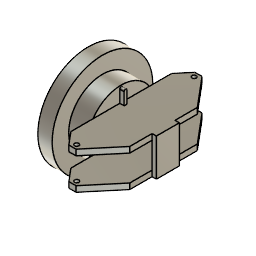
model (Autodesk Fusion 360 archive; units mm, degrees)
design "jaw 6"
part number: 2025-10-28-00-25-30-130
part number: 2025-10-28-00-26-21-145
Autodesk Fusion 360 part; units mm, degrees
sketch "Sketch1" plane through (0, 0, 0) normal (1, 0, 0) x (0, 1, 0)
  circle A0 centre (0, 0) radius 35
  dimension "d1" = 70
  constraint coincident A0.centre origin
  measures "d1" diameter of A0
extrude "Extrude1" add sketch "Sketch1" along normal blind 10 in component "Component"
sketch "Sketch2" plane through (10, 0, 0) normal (1, 0, 0) x (0, 1, 0)
  circle A0 centre (0, 0) radius 35
  circle A1 centre (0, 0) radius 23.5
  dimension "d4" = 47
  constraint concentric A0 A1
  measures "d4" diameter of A1
extrude "Extrude2" add sketch "Sketch2" along normal blind 13 contours A1 in component "Component"
ref_plane "WorkPlane1" through (0, 0, 13) normal (0, 0, 1) x (1, 0, 0)
sketch "Sketch3" plane through (0, 0, 13) normal (0, 0, 1) x (1, 0, 0)
  line L0 (23, 0) -> (23, -35)
  line L1 (23, -35) -> (23, -42)
  line L2 (23, -35) -> (30.3921, -43.8095)
  line L3 (30.3921, -43.8095) -> (35.3921, -43.8095)
  line L4 (23, 0) -> (63, 0)
  line L5 (23, -23.5) -> (65.3695, -23.5)
  line L6 (35.3921, -43.8095) -> (52.4338, -23.5)
  line L7 (35.3921, -43.8095) -> (49, -43.8095)
  line L8 (52.4338, -23.5) -> (52.4338, 0)
  line L9 (35.3921, 43.8095) -> (52.4338, 23.5)
  line L10 (30.3921, 43.8095) -> (35.3921, 43.8095)
  line L11 (23, 35) -> (30.3921, 43.8095)
  line L12 (23, 0) -> (23, 35)
  line L13 (23, 0) -> (63, 0)
  line L14 (52.4338, 23.5) -> (52.4338, 0)
  dimension "d8" = 35
  dimension "d9" = 11.5
  dimension "d10" = 40
  dimension "d11" = 5
  dimension "d12" = 50
  constraint vertical L0
  constraint parallel L0 L1
  constraint horizontal L3
  constraint perpendicular L0 L4
  constraint coincident L0 L5.start
  constraint perpendicular L0 L5
  constraint coincident L5 L6.end
  constraint parallel L3 L7
  constraint coincident L4 L8.end
  constraint perpendicular L4 L8
  constraint symmetric L0.start L4 L12.start
  constraint symmetric L0.end L4 L11.start
  constraint symmetric L2.end L4 L10.start
  constraint symmetric L3.end L4 L9.start
  constraint symmetric L13.end L4 L4.end
  constraint symmetric L4 L6.end L9.end
  constraint symmetric L4 L8.end L14.end
  measures "d8" distance of L0.start L0.end
  measures "d9" distance of L0.end L2.end
  measures "d10" angle of L1 L2
  measures "d11" distance of L2.end L3.end
  measures "d12" angle of L6 L7
extrude "Extrude3" add sketch "Sketch3" against normal blind 4 in component "Component"
sketch "Sketch4" plane through (0, 0, 13) normal (0, 0, 1) x (-1, 0, 0)
  line L0 (-23, -35) -> (-23, -19.5768)
  line L1 (-23, -19.5768) -> (-23, 19.5768)
  line L2 (-23, 19.5768) -> (-23, 35)
  line L3 (-23, 35) -> (-30.3921, 43.8095)
  line L4 (-30.3921, 43.8095) -> (-35.3921, 43.8095)
  line L5 (-35.3921, 43.8095) -> (-52.4338, 23.5)
  line L6 (-52.4338, 23.5) -> (-52.4338, -23.5)
  line L7 (-52.4338, -23.5) -> (-35.3921, -43.8095)
  line L8 (-35.3921, -43.8095) -> (-30.3921, -43.8095)
  line L9 (-30.3921, -43.8095) -> (-23, -35)
  line L10 (-32.8921, 43.8095) -> (-32.8921, 40.8095)
  circle A0 centre (-32.8921, 40.8095) radius 1.5
  dimension "d15" = 3
  dimension "d16" = 3
  constraint midpoint L4 L10.start
  constraint perpendicular L4 L10
  constraint coincident L10.end A0.centre
  measures "d15" distance of L10.start L10.end
  measures "d16" diameter of A0
extrude "Extrude4" cut sketch "Sketch4" against normal blind 11.5 contours A0 in component "Component"
mirror "Mirror1" about plane through (0, 0, 0) normal (0, 1, 0) of "Extrude4" in component "Component"
mirror "Mirror2" about plane through (0, 0, 0) normal (0, 0, 1) of "Extrude3", "Extrude4", "Mirror1" in component "Component"
sketch "Sketch5" plane through (23, 0, 0) normal (1, 0, 0) x (0, 1, 0)
  line L0 (-19.5768, 13) -> (19.5768, 13)
  arc A0 (19.5768, 13) -> (-19.5768, 13) centre (0, 0) ccw
  line L1 (0, 13) -> (0, 23.5)
  line L2 (0, 13) -> (-1, 13)
  line L3 (-1, 13) -> (-1, 13.5345)
  line L4 (-1, 13.5345) -> (-1, 22.5345)
  line L5 (-1, 22.5345) -> (1, 22.5345)
  line L6 (1, 22.5345) -> (1, 13)
  dimension "d23" = 1
  dimension "d24" = 9
  dimension "d25" = 2
  constraint midpoint L0 L1.start
  constraint midpoint A0 L1.end
  constraint perpendicular L1 L2
  constraint perpendicular L2 L3
  constraint perpendicular L2 L4
  constraint perpendicular L1 L5
  constraint coincident L0 L6.end
  constraint perpendicular L0 L6
  measures "d23" distance of L1.start L2.end
  measures "d24" distance of L3.end L4.end
  measures "d25" distance of L4.end L5.end
extrude "Extrude5" add sketch "Sketch5" along normal blind 3 contours L0 L1 L2 L3 L4 L5 | L0 L1 L5 L6 in component "Component"
fillet "Fillet1" radius 1 2 edges at (24.5, 1, 22.5345) (24.5, -1, 22.5345) in component "Component"
mirror "Mirror3" about plane through (0, 0, 0) normal (0, 0, 1) of "Extrude5", "Fillet1" in component "Component"
sketch "Sketch6" plane through (52.4338, 0, 0) normal (1, 0, 0) x (0, 1, 0)
  line L0 (23.5, 13) -> (-23.5, 13)
  line L1 (-23.5, 13) -> (-23.5, 9)
  line L2 (-23.5, 9) -> (23.5, 9)
  line L3 (23.5, 9) -> (23.5, 13)
  line L4 (8, -13) -> (-8, -13)
  line L5 (-8, -13) -> (-8, 13)
  line L6 (-8, 13) -> (8, 13)
  line L7 (8, 13) -> (8, -13)
  line L8 (8, -13) -> (-8, 13) construction
  line L9 (-8, -13) -> (8, 13) construction
  dimension "d32" = 16
  dimension "d33" = 26
  constraint horizontal L4
  constraint perpendicular L4 L5
  constraint parallel L4 L6
  constraint parallel L5 L7
  constraint coincident L8 origin
  constraint coincident L9 origin
  measures "d32" distance of L5.end L6.end
  measures "d33" distance of L4.end L5.end
extrude "Extrude6" add sketch "Sketch6" along normal blind 3 contours L0 L2 L5 L6 L7 | L2 L4 L5 L7 in component "Component"
sketch "Sketch7" plane through (0, 0, 0) normal (-1, 0, 0) x (0, -1, 0)
  circle A0 centre (0, 0) radius 35
  circle A1 centre (0, 0) radius 10
  dimension "d36" = 20
  constraint coincident A0.centre A1.centre
  measures "d36" diameter of A1
extrude "Extrude7" cut sketch "Sketch7" against normal blind 10 contours A1 in component "Component"
component "Component" placed x (1, 0, 0) y (0, 1, 0) z (0, 0, 1) at (0, 0, 0)
equation "d4 = 23.5 * 2 mm"

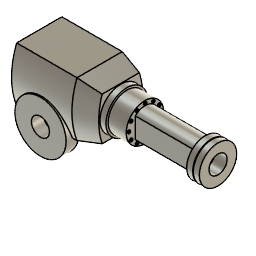
design "part 3"
part number: 2025-10-27-21-08-31-272
part number: 2025-10-27-21-14-58-809
Autodesk Fusion 360 part; units mm, degrees
sketch "Sketch1" plane through (0, 0, 0) normal (1, 0, 0) x (0, 1, 0)
  line L0 (0, 0) -> (0, 45)
  line L1 (0, 0) -> (0, -45)
  line L2 (0, 45) -> (37.5, 45)
  line L3 (0, 45) -> (-37.5, 45)
  line L4 (0, -45) -> (-37.5, -45)
  arc A0 (-37.5, 45) -> (-37.5, -45) centre (79.119, 0) ccw
  line L5 (0, -45) -> (37.5, -45)
  arc A1 (37.5, -45) -> (37.5, 45) centre (-79.119, 0) ccw
  dimension "d2" = 45
  dimension "d3" = 37.5
  dimension "d4" = 37.5
  dimension "d5" = 37.5
  dimension "d6" = 37.5
  dimension "d7" = 125
  dimension "d8" = 125
  constraint coincident L0.start L1.start
  constraint vertical L0
  constraint parallel L0 L1
  constraint perpendicular L0 L2
  constraint perpendicular L0 L3
  constraint perpendicular L1 L4
  constraint perpendicular L1 L5
  measures "d2" distance of L0.start L1.end
  measures "d3" distance of L0.end L2.end
  measures "d4" distance of L0.end L3.end
  measures "d5" distance of L1.end L4.end
  measures "d6" distance of L1.end L5.end
  measures "d7" radius of A1
  measures "d8" radius of A0
extrude "Extrude1" add sketch "Sketch1" along normal blind 100 in component "jaw 3"
extrude "Extrude2" add 1 faces at (100, -15.1807, 3.0661) along direction (1, 0, 0) blind 35 draft -15 in component "jaw 3"
sketch "Sketch2" plane through (135, 0, 0) normal (1, 0, 0) x (0, 1, 0)
  line L0 (-30.8786, -35.6218) -> (30.8786, -35.6218)
  arc A0 (30.8786, -35.6218) -> (30.8786, 35.6218) centre (-79.119, 0) ccw
  line L1 (30.8786, 35.6218) -> (-30.8786, 35.6218)
  arc A1 (-30.8786, 35.6218) -> (-30.8786, -35.6218) centre (79.119, 0) ccw
  circle A2 centre (0, 0) radius 34.5
  dimension "d13" = 69
  constraint coincident A2.centre origin
  measures "d13" diameter of A2
extrude "Extrude3" add sketch "Sketch2" along normal blind 10 contours A2 in component "jaw 3"
sketch "Sketch3" plane through (145, 0, 0) normal (1, 0, 0) x (0, 1, 0)
  circle A0 centre (0, 0) radius 34.5
  circle A1 centre (0, 0) radius 31
  dimension "d16" = 62
  constraint coincident A0.centre A1.centre
  measures "d16" diameter of A1
extrude "Extrude4" add sketch "Sketch3" along normal blind 30 contours A1 in component "jaw 3"
sketch "Sketch4" plane through (175, 0, 0) normal (1, 0, 0) x (0, 1, 0)
  circle A0 centre (0, 0) radius 31
  line L0 (0, 0) -> (27, 0)
  circle A1 centre (27, 0) radius 2.5
  circle A2 centre (27, 0) radius 1.5
  dimension "d19" = 27
  dimension "d20" = 5
  dimension "d21" = -1
  constraint coincident A0.centre L0.start
  constraint horizontal L0
  constraint coincident L0.end A1.centre
  measures "d19" distance of A0.centre L0.end
  measures "d20" diameter of A1
extrude "Extrude5" add sketch "Sketch4" along normal blind 1 contours A1 in component "jaw 3"
pattern_circular "C-Pattern1" count 12 over 360 about axis through (175, 0, 0) along (1, 0, 0) of "Extrude5" in component "jaw 3"
sketch "Sketch5" plane through (175, 0, 0) normal (1, 0, 0) x (0, 1, 0)
  circle A0 centre (13.5, -23.3827) radius 2.5
  circle A1 centre (-13.5, -23.3827) radius 2.5
  circle A2 centre (-27, 0) radius 2.5
  circle A3 centre (-13.5, 23.3827) radius 2.5
  circle A4 centre (13.5, 23.3827) radius 2.5
  circle A5 centre (27, 0) radius 2.5
  circle A6 centre (0, 0) radius 31
  circle A7 centre (23.3827, 13.5) radius 2.5
  circle A8 centre (0, 27) radius 2.5
  circle A9 centre (-23.3827, 13.5) radius 2.5
  circle A10 centre (-23.3827, -13.5) radius 2.5
  circle A11 centre (0, -27) radius 2.5
  circle A12 centre (23.3827, -13.5) radius 2.5
  line L0 (0, 0) -> (16, 0)
  line L1 (0, 0) -> (0, -6)
  line L2 (16, 0) -> (16, -17)
  line L3 (16, 0) -> (16, 17)
  line L4 (0, 0) -> (-16, 0)
  line L5 (-16, 0) -> (-16, -17)
  line L6 (-16, 0) -> (-16, 17)
  arc A13 (16, 17) -> (-16, 17) centre (0, 1.9003) ccw
  arc A14 (-16, -17) -> (16, -17) centre (0, -1.9003) ccw
  dimension "d26" = 16
  dimension "d27" = 17
  dimension "d28" = 17
  dimension "d29" = 16
  dimension "d30" = 17
  dimension "d31" = 17
  dimension "d32" = 22
  dimension "d33" = 22
  constraint coincident A6.centre L0.start
  constraint horizontal L0
  constraint perpendicular L0 L1
  constraint perpendicular L0 L2
  constraint perpendicular L0 L3
  constraint perpendicular L1 L4
  constraint perpendicular L4 L5
  constraint perpendicular L4 L6
  measures "d26" distance of A6.centre L0.end
  measures "d27" distance of L0.end L2.end
  measures "d28" distance of L0.end L3.end
  measures "d29" distance of A6.centre L4.end
  measures "d30" distance of L4.end L5.end
  measures "d31" distance of L4.end L6.end
  measures "d32" radius of A13
  measures "d33" radius of A14
extrude "Extrude6" add sketch "Sketch5" along normal blind 100 contours L0 L3 L4 L6 A13 | L0 L2 L4 L5 A14 in component "jaw 3"
sketch "Sketch6" plane through (275, 0, 0) normal (1, 0, 0) x (0, 1, 0)
  line L0 (-16, 17) -> (-16, -17)
  arc A0 (-16, -17) -> (16, -17) centre (0, -1.9003) ccw
  line L1 (16, -17) -> (16, 17)
  arc A1 (16, 17) -> (-16, 17) centre (0, 1.9003) ccw
  circle A2 centre (0, 0) radius 30.9959
  constraint coincident A2.centre origin
extrude "Extrude7" add sketch "Sketch6" along normal blind 10 contours L0 A0 L1 A1 | A2 in component "jaw 3"
sketch "Sketch7" plane through (285, 0, 0) normal (1, 0, 0) x (0, 1, 0)
  circle A0 centre (0, 0) radius 30.9959
  circle A1 centre (0, 0) radius 29.9959
  dimension "d38" = -1
extrude "Extrude8" add sketch "Sketch7" along normal blind 1 contours A1 in component "jaw 3"
sketch "Sketch8" plane through (286, 0, 0) normal (1, 0, 0) x (0, 1, 0)
  circle A0 centre (0, 0) radius 29.9959
  circle A1 centre (0, 0) radius 31.0015
  constraint coincident A0.centre A1.centre
extrude "Extrude9" add sketch "Sketch8" along normal blind 10 contours A0 | A1 in component "jaw 3"
ref_plane "WorkPlane1" through (0, -37.5, 45) normal (0, -1, 0) x (1, 0, 0)
sketch "Sketch9" plane through (0, -37.5, 0) normal (0, -1, 0) x (-1, 0, 0)
  circle A0 centre (-50, 45) radius 42.5
  dimension "d43" = 85
  measures "d43" diameter of A0
extrude "Extrude10" add sketch "Sketch9" along normal mid plane 21 in component "jaw 3"
sketch "Sketch10" plane through (0, -27, 0) normal (0, 1, 0) x (-1, 0, 0)
  line L0 (-7.5, -45) -> (-92.5, -45)
  arc A0 (-92.5, -45) -> (-7.5, -45) centre (-50, -45) ccw
  line L1 (-50, -45) -> (-50, -75)
  line L2 (-70, -45) -> (-70, -75.0144)
  line L3 (-30, -45) -> (-30, -75.0144)
  arc A1 (-70, -75.0144) -> (-30, -75.0144) centre (-50, -52.6537) ccw
  dimension "d46" = 30
  dimension "d47" = 20
  dimension "d48" = -20
  dimension "d49" = 30
  constraint coincident A0.centre L1.start
  constraint perpendicular L0 L1
  measures "d46" distance of A0.centre L1.end
  measures "d49" radius of A1
extrude "Extrude11" add sketch "Sketch10" along normal blind 35 contours L0 L2 L3 A1 in component "jaw 3"
sketch "Sketch11" plane through (70, 0, 0) normal (1, 0, 0) x (0, 1, 0)
  line L0 (-27, -45) -> (-27, -75.0144)
  line L1 (-27, -75.0144) -> (8, -75.0144)
  line L2 (8, -75.0144) -> (8, -45)
  line L3 (8, -45) -> (-27, -45)
  line L4 (8, -45) -> (33, -45)
  line L5 (8, -45) -> (8, -87)
  arc A0 (8, -87) -> (33, -45) centre (-21.8393, -40.7981) ccw
  dimension "d52" = 25
  dimension "d53" = 42
  dimension "d54" = 55
  constraint coincident L2.end L3.start
  constraint perpendicular L2 L4
  constraint perpendicular L1 L5
  measures "d52" distance of L2.end L4.end
  measures "d53" distance of L2.end L5.end
  measures "d54" radius of A0
extrude "Extrude12" add sketch "Sketch11" against normal blind 40 contours L2 L4 L5 A0 in component "jaw 3"
extrude "Extrude13" cut 1 faces at (50, 8, -85.5512) along direction (0, 1, 0) blind 90 in component "jaw 3"
sketch "Sketch12" plane through (296, 0, 0) normal (1, 0, 0) x (0, 1, 0)
  circle A0 centre (0, 0) radius 31.0015
  circle A1 centre (0, 0) radius 15
  dimension "d59" = 30
  constraint coincident A0.centre A1.centre
  measures "d59" diameter of A1
extrude "Extrude14" cut sketch "Sketch12" against normal blind 20 contours A1 in component "jaw 3"
sketch "Sketch13" plane through (0, -48, 0) normal (0, -1, 0) x (1, 0, 0)
  circle A0 centre (50, -45) radius 42.5
  circle A1 centre (50, -45) radius 15
  dimension "d62" = 30
  constraint concentric A0 A1
  measures "d62" diameter of A1
extrude "Extrude15" cut sketch "Sketch13" against normal blind 20 contours A1 in component "jaw 3"
component "jaw 3" placed x (1, 0, 0) y (0, 1, 0) z (0, 0, 1) at (0, 0, 0)
equation "d44 = ( 21 / 2 ) * 1 mm"

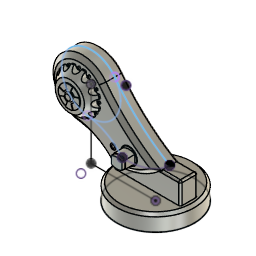
design "Jaw"
part number: 2025-10-27-12-31-22-567
part number: 2025-10-27-12-32-54-316
Autodesk Fusion 360 part; units mm, degrees
sketch "Sketch1" plane through (0, 0, 0) normal (0, 0, 1) x (1, 0, 0)
  circle A0 centre (0, 0) radius 90
  dimension "d1" = 180
  constraint coincident A0.centre origin
  measures "d1" diameter of A0
extrude "Extrude1" add sketch "Sketch1" along normal blind 37 in component "Component"
chamfer "Chamfer1" distance 6 angle 45 1 edges at (-83.9095, -32.5454, 37) in component "Component"
sketch "Sketch2" plane through (0, 0, 37) normal (0, 0, 1) x (-1, 0, 0)
  circle A0 centre (0, 0) radius 84
  line L0 (-77.5, 20) -> (77.5, 20)
  line L1 (77.5, 20) -> (77.5, -20)
  line L2 (77.5, -20) -> (-77.5, -20)
  line L3 (-77.5, -20) -> (-77.5, 20)
  line L4 (-77.5, 20) -> (77.5, -20) construction
  line L5 (77.5, 20) -> (-77.5, -20) construction
  dimension "d5" = 155
  dimension "d6" = 40
  constraint horizontal L0
  constraint perpendicular L0 L1
  constraint parallel L0 L2
  constraint parallel L1 L3
  constraint coincident L4 A0.centre
  constraint coincident L5 A0.centre
  constraint coincident A0.centre origin
  measures "d5" distance of L1.end L2.end
  measures "d6" distance of L0.end L1.end
  measures "d9" distance of L2.end
  measures "d10" distance of L2.end
extrude "Extrude2" add sketch "Sketch2" along normal blind 50 contours L0 L1 L2 L3 in component "Component"
sketch "Sketch3" plane through (0, -20, 0) normal (0, -1, 0) x (1, 0, 0)
  line L0 (-77.5, 37) -> (77.5, 37)
  line L1 (77.5, 37) -> (77.5, 87)
  line L2 (77.5, 87) -> (-77.5, 87)
  line L3 (-77.5, 87) -> (-77.5, 37)
  line L4 (-77.5, 87) -> (32.5, 87)
  line L5 (-77.5, 87) -> (-77.5, 48)
  arc A0 (-77.5, 48) -> (32.5, 87) centre (-68.6761, 197.7402) ccw
  dimension "d9" = 110
  dimension "d10" = 39
  dimension "d11" = 150
  constraint coincident L2.end L3.start
  constraint coincident L2 L4.end
  constraint coincident L3 L5.end
  measures "d9" distance of L2.end L4.end
  measures "d10" distance of L2.end L5.end
  measures "d11" radius of A0
extrude "Extrude3" cut sketch "Sketch3" against normal blind 230 contours L2 L3 L4 L5 A0 in component "Component"
sketch "Sketch4" plane through (0, 0, 0) normal (0, 1, 0) x (1, 0, 0)
  line L0 (0, 0) -> (-150, 0)
  circle A0 centre (-150, -160) radius 68.5
  arc A1 (32.5, -87) -> (-95.2795, -201.2057) centre (256.2101, -465.8849) ccw
  arc A2 (-158.3154, -92.0066) -> (-77.5, -48) centre (-173.4894, 32.069) ccw
  arc A3 (32.5, -87) -> (-77.5, -48) centre (-68.6761, -197.7402) ccw
  point P0 (-77.5, -48)
  point P1 (32.5, -87)
  dimension "d14" = 150
  dimension "d15" = 160
  dimension "d16" = 137
  dimension "d17" = 440
  dimension "d18" = 125
  dimension "d19" = 150
  constraint coincident L0.start origin
  constraint horizontal L0
  constraint tangent A0 A1
  constraint tangent A0 A2
  constraint coincident P0 A2.end
  constraint coincident P1 A1.start
  constraint coincident A0 A1.end
  constraint coincident A0 A2.start
  measures "d14" distance of L0.start L0.end
  measures "d15" distance of L0.end A0.centre
  measures "d16" diameter of A0
  measures "d17" radius of A1
  measures "d18" radius of A2
  measures "d19" radius of A3
extrude "Extrude4" add sketch "Sketch4" along normal mid plane 40 in component "Component"
sketch "Sketch5" plane through (0, 0, 0) normal (0, 1, 0) x (1, 0, 0)
  circle A0 centre (-150, -160) radius 68.5
  arc A1 (32.5, -87) -> (-95.2795, -201.2057) centre (256.2101, -465.8849) ccw
  arc A2 (-158.3154, -92.0066) -> (-77.5, -48) centre (-173.4894, 32.069) ccw
  arc A3 (32.5, -87) -> (-77.5, -48) centre (-68.6761, -197.7402) ccw
  line L0 (-150, -160) -> (-150, 0)
  constraint coincident A0.centre L0.start
  constraint vertical L0
sketch "Sketch6" plane through (0, -20, 0) normal (0, -1, 0) x (1, 0, 0)
  line L0 (-77.5, 48) -> (-77.5, 37)
  line L1 (-77.5, 37) -> (77.5, 37)
  line L2 (77.5, 37) -> (77.5, 87)
  line L3 (77.5, 87) -> (32.5, 87)
  arc A0 (-95.2795, 201.2057) -> (32.5, 87) centre (256.2101, 465.8849) ccw
  arc A1 (-95.2795, 201.2057) -> (-158.3154, 92.0066) centre (-150, 160) ccw
  arc A2 (-77.5, 48) -> (-158.3154, 92.0066) centre (-173.4894, -32.069) ccw
  arc A3 (-95.2795, 201.2057) -> (32.5, 87) centre (256.2101, 465.8849) ccw
  arc A4 (-77.5, 48) -> (-158.3154, 92.0066) centre (-173.4894, -32.069) ccw
  circle A5 centre (-150, 160) radius 68.5
  arc A6 (-77.5, 48) -> (32.5, 87) centre (-68.6761, 197.7402) ccw
extrude "Extrude5" add sketch "Sketch6" along normal blind 7.5 draft -55 contours A0 A2 A3 A4 A5 A6 | A1 A5 in component "Component"
sketch "Sketch7" plane through (0, -27.5, 0) normal (0, -1, 0) x (1, 0, 0)
  arc A0 (-103.8359, 194.7625) -> (-157.0151, 102.6385) centre (-150, 160) ccw
  arc A1 (-72.4228, 58.5017) -> (-157.0151, 102.6385) centre (-173.4894, -32.069) ccw
  arc A2 (-72.4228, 58.5017) -> (14.1053, 85.7195) centre (-68.6761, 197.7402) ccw
  arc A3 (-103.8359, 194.7625) -> (14.1053, 85.7195) centre (256.2101, 465.8849) ccw
  circle A4 centre (-150, 160) radius 50
  dimension "d24" = 100
  constraint concentric A0 A4
  measures "d24" diameter of A4
extrude "Extrude6" add sketch "Sketch7" along normal blind 3 contours A4 in component "Component"
extrude "Extrude7" add 1 faces at (-167.3965, -30.5, 167.9656) along direction (0, -1, 0) blind 19 draft -40 in component "Component"
sketch "Sketch8" plane through (0, -49.5, 0) normal (0, -1, 0) x (1, 0, 0)
  circle A0 centre (-150, 160) radius 34.0571
  line L0 (-150, 160) -> (-150, 210)
  arc A1 (-158.9635, 209.19) -> (-150, 201) centre (-150, 210) ccw
  circle A2 centre (-150, 160) radius 50
  arc A3 (-150, 201) -> (-141.0365, 209.19) centre (-150, 210) ccw
  dimension "d29" = 9
  dimension "d30" = 9
  constraint coincident A0.centre L0.start
  constraint vertical L0
  constraint coincident L0 A1.end
  constraint coincident A1.start A2
  constraint symmetric L0 A1.end A3.start
  constraint symmetric L0 A1.start A3.end
  constraint symmetric L0 A1 A3
  measures "d29" distance of L0.end A1.end
  measures "d30" radius of A1
extrude "Extrude8" cut sketch "Sketch8" against normal up to surface (22 mm away) contours L0 A1 A2 | L0 A2 A3 in component "Component"
sketch "Sketch9" plane through (0, -27.5, 0) normal (0, -1, 0) x (1, 0, 0)
  arc A0 (-158.9635, 209.19) -> (-141.0365, 209.19) centre (-150, 160) ccw
  arc A1 (-158.9635, 209.19) -> (-141.0365, 209.19) centre (-150, 210) ccw
  arc A2 (-103.8359, 194.7625) -> (-157.0151, 102.6385) centre (-150, 160) ccw
  arc A3 (-72.4228, 58.5017) -> (-157.0151, 102.6385) centre (-173.4894, -32.069) ccw
  arc A4 (-72.4228, 58.5017) -> (14.1053, 85.7195) centre (-68.6761, 197.7402) ccw
  arc A5 (-103.8359, 194.7625) -> (14.1053, 85.7195) centre (256.2101, 465.8849) ccw
  line L0 (-150, 201) -> (-150, 217.7889)
  circle A6 centre (-150, 207) radius 3
  circle A7 centre (-150, 207) radius 1.6
  dimension "d33" = 6
  dimension "d34" = -1.4
  constraint midpoint A1 L0.start
  constraint coincident A2 L0.end
  constraint vertical L0
  constraint coincident L0 A6.centre
  measures "d33" diameter of A6
extrude "Extrude9" add sketch "Sketch9" along normal blind 3 contours L0 A6 A7 | L0 A6 A7 in component "Component"
pattern_circular "C-Pattern1" count 12 over 360 about axis through (-150, -49.5, 160) along (0, 1, 0) of "Extrude8", "Extrude9" in component "Component"
sketch "Sketch10" plane through (0, -49.5, 0) normal (0, -1, 0) x (1, 0, 0)
  circle A0 centre (-150, 160) radius 34.0571
  circle A1 centre (-150, 160) radius 13
  circle A2 centre (-150, 160) radius 25
  dimension "d39" = 26
  dimension "d40" = 50
  constraint concentric A0 A1
  constraint concentric A1 A2
  measures "d39" diameter of A1
  measures "d40" diameter of A2
extrude "Extrude10" add sketch "Sketch10" along normal blind 1 contours A1 | A2 in component "Component"
sketch "Sketch11" plane through (0, -50.5, 0) normal (0, -1, 0) x (1, 0, 0)
  circle A0 centre (-150, 160) radius 25
  circle A1 centre (-150, 160) radius 12.5
  line L0 (-154.799, 171.5421) -> (-159.0764, 183.2942)
  line L1 (-146.3157, 171.9447) -> (-141.6715, 183.5719)
  line L2 (-161.5421, 155.201) -> (-173.2942, 150.9236)
  line L3 (-161.9447, 163.6843) -> (-173.5719, 168.3285)
  line L4 (-145.201, 148.4579) -> (-140.9236, 136.7058)
  line L5 (-153.6843, 148.0553) -> (-158.3285, 136.4281)
  line L6 (-138.4579, 164.799) -> (-126.7058, 169.0764)
  line L7 (-138.0553, 156.3157) -> (-126.4281, 151.6715)
  dimension "d43" = 25
  dimension "d46" = 360
  constraint concentric A0 A1
  constraint coincident A1 L0.start
  constraint coincident A0 L0.end
  constraint coincident A0 L1.end
  constraint coincident A1 L1.start
  measures "d43" diameter of A1
extrude "Extrude11" add sketch "Sketch11" along normal blind 1 contours A0 A1 L6 L7 | A0 A1 L0 L1 | A1 | A0 A1 L4 L5 | A0 A1 L2 L3 in component "Component"
sketch "Sketch12" plane through (0, -51.5, 0) normal (0, -1, 0) x (1, 0, 0)
  arc A0 (-145.201, 148.4579) -> (-138.0553, 156.3157) centre (-150, 160) ccw
  line L0 (-138.0553, 156.3157) -> (-126.4281, 151.6715)
  arc A1 (-126.4281, 151.6715) -> (-126.7058, 169.0764) centre (-150, 160) ccw
  line L1 (-126.7058, 169.0764) -> (-138.4579, 164.799)
  arc A2 (-138.4579, 164.799) -> (-146.3157, 171.9447) centre (-150, 160) ccw
  line L2 (-146.3157, 171.9447) -> (-141.6715, 183.5719)
  arc A3 (-141.6715, 183.5719) -> (-159.0764, 183.2942) centre (-150, 160) ccw
  line L3 (-159.0764, 183.2942) -> (-154.799, 171.5421)
  arc A4 (-154.799, 171.5421) -> (-161.9447, 163.6843) centre (-150, 160) ccw
  line L4 (-161.9447, 163.6843) -> (-173.5719, 168.3285)
  arc A5 (-173.5719, 168.3285) -> (-173.2942, 150.9236) centre (-150, 160) ccw
  line L5 (-173.2942, 150.9236) -> (-161.5421, 155.201)
  arc A6 (-161.5421, 155.201) -> (-153.6843, 148.0553) centre (-150, 160) ccw
  line L6 (-153.6843, 148.0553) -> (-158.3285, 136.4281)
  arc A7 (-158.3285, 136.4281) -> (-140.9236, 136.7058) centre (-150, 160) ccw
  line L7 (-140.9236, 136.7058) -> (-145.201, 148.4579)
  circle A8 centre (-150, 160) radius 9.5
  dimension "d49" = 19
  constraint concentric A0 A8
  measures "d49" diameter of A8
extrude "Extrude12" add sketch "Sketch12" along normal blind 3 draft -45 contours A8 in component "Component"
sketch "Sketch13" plane through (0, -27.5, 0) normal (0, -1, 0) x (1, 0, 0)
  circle A0 centre (-190.7032, 183.5) radius 3
  circle A1 centre (-190.7032, 136.5) radius 3
  circle A2 centre (-150, 113) radius 3
  circle A3 centre (-109.2968, 136.5) radius 3
  circle A4 centre (-109.2968, 183.5) radius 3
  circle A5 centre (-150, 207) radius 3
  arc A6 (-133.1676, 207.0815) -> (-141.0365, 209.19) centre (-150, 160) ccw
  arc A7 (-133.1676, 207.0815) -> (-117.6424, 198.118) centre (-125, 203.3013) ccw
  arc A8 (-111.8819, 192.3576) -> (-117.6424, 198.1181) centre (-150, 160) ccw
  arc A9 (-111.8819, 192.3576) -> (-102.9185, 176.8324) centre (-106.6987, 185) ccw
  arc A10 (-100.81, 168.9635) -> (-102.9185, 176.8324) centre (-150, 160) ccw
  arc A11 (-100.81, 168.9635) -> (-100.81, 151.0365) centre (-100, 160) ccw
  arc A12 (-102.9185, 143.1676) -> (-100.81, 151.0365) centre (-150, 160) ccw
  arc A13 (-102.9185, 143.1676) -> (-111.882, 127.6424) centre (-106.6987, 135) ccw
  arc A14 (-117.6424, 121.8819) -> (-111.8819, 127.6424) centre (-150, 160) ccw
  arc A15 (-117.6424, 121.8819) -> (-133.1676, 112.9185) centre (-125, 116.6987) ccw
  arc A16 (-141.0365, 110.81) -> (-133.1676, 112.9185) centre (-150, 160) ccw
  arc A17 (-141.0365, 110.81) -> (-158.9635, 110.81) centre (-150, 110) ccw
  arc A18 (-166.8324, 112.9185) -> (-158.9635, 110.81) centre (-150, 160) ccw
  arc A19 (-166.8324, 112.9185) -> (-182.3576, 121.882) centre (-175, 116.6987) ccw
  arc A20 (-188.1181, 127.6424) -> (-182.3576, 121.8819) centre (-150, 160) ccw
  arc A21 (-188.1181, 127.6424) -> (-197.0815, 143.1676) centre (-193.3013, 135) ccw
  arc A22 (-199.19, 151.0365) -> (-197.0815, 143.1676) centre (-150, 160) ccw
  arc A23 (-199.19, 151.0365) -> (-199.19, 168.9635) centre (-200, 160) ccw
  arc A24 (-197.0815, 176.8324) -> (-199.19, 168.9635) centre (-150, 160) ccw
  arc A25 (-197.0815, 176.8324) -> (-188.118, 192.3576) centre (-193.3013, 185) ccw
  arc A26 (-182.3576, 198.1181) -> (-188.1181, 192.3576) centre (-150, 160) ccw
  arc A27 (-182.3576, 198.1181) -> (-166.8324, 207.0815) centre (-175, 203.3013) ccw
  arc A28 (-158.9635, 209.19) -> (-166.8324, 207.0815) centre (-150, 160) ccw
  arc A29 (-158.9635, 209.19) -> (-141.0365, 209.19) centre (-150, 210) ccw
  arc A30 (-103.8359, 194.7625) -> (-157.0151, 102.6385) centre (-150, 160) ccw
  arc A31 (-72.4228, 58.5017) -> (-157.0151, 102.6385) centre (-173.4894, -32.069) ccw
  arc A32 (-72.4228, 58.5017) -> (14.1053, 85.7195) centre (-68.6761, 197.7402) ccw
  arc A33 (-103.8359, 194.7625) -> (14.1053, 85.7195) centre (256.2101, 465.8849) ccw
  circle A34 centre (-126.5, 200.7032) radius 3
  circle A35 centre (-103, 160) radius 3
  circle A36 centre (-126.5, 119.2968) radius 3
  circle A37 centre (-173.5, 119.2968) radius 3
  circle A38 centre (-197, 160) radius 3
  circle A39 centre (-173.5, 200.7032) radius 3
  line L0 (-47.7688, 96.5857) -> (-20.7688, 96.5857)
  line L1 (-20.7688, 96.5857) -> (-20.7688, 77.5857)
  line L2 (-20.7688, 77.5857) -> (-47.7688, 77.5857)
  line L3 (-47.7688, 77.5857) -> (-47.7688, 96.5857)
  arc A40 (-20.7688, 96.5857) -> (-47.7688, 96.5857) centre (-34.2688, 73.203) ccw
  arc A41 (-47.7688, 77.5857) -> (-20.7688, 77.5857) centre (-34.2688, 100.9684) ccw
  dimension "d52" = 27
  dimension "d53" = 19
  dimension "d54" = 27
  dimension "d55" = 27
  constraint horizontal L0
  constraint vertical L1
  constraint horizontal L2
  constraint vertical L3
  measures "d52" distance of L0.start L0.end
  measures "d53" distance of L0.start L2.end
  measures "d54" radius of A40
  measures "d55" radius of A41
extrude "Extrude13" add sketch "Sketch13" along normal blind 22 contours L0 A40 | L0 L1 L2 L3 | L2 A41 in component "Component"
sketch "Sketch14" plane through (0, -49.5, 0) normal (0, -1, 0) x (1, 0, 0)
  arc A0 (-20.7688, 96.5857) -> (-47.7688, 96.5857) centre (-34.2688, 73.203) ccw
  line L0 (-47.7688, 96.5857) -> (-47.7688, 77.5857)
  arc A1 (-47.7688, 77.5857) -> (-20.7688, 77.5857) centre (-34.2688, 100.9684) ccw
  line L1 (-20.7688, 77.5857) -> (-20.7688, 96.5857)
  arc A2 (-46.6178, 78.26) -> (-21.9198, 78.26) centre (-34.2688, 100.9684) ccw
  line L2 (-21.9198, 78.26) -> (-21.9198, 95.9115)
  arc A3 (-21.9198, 95.9115) -> (-46.6178, 95.9115) centre (-34.2688, 73.203) ccw
  line L3 (-46.6178, 95.9115) -> (-46.6178, 78.26)
  dimension "d58" = -1.151
extrude "Extrude14" add sketch "Sketch14" along normal blind 7 contours A2 L2 A3 L3 in component "Component"
sketch "Sketch15" plane through (0, -56.5, 0) normal (0, -1, 0) x (1, 0, 0)
  line L0 (-46.6178, 95.9115) -> (-46.6178, 78.26)
  arc A0 (-46.6178, 78.26) -> (-21.9198, 78.26) centre (-34.2688, 100.9684) ccw
  line L1 (-21.9198, 78.26) -> (-21.9198, 95.9115)
  arc A1 (-21.9198, 95.9115) -> (-46.6178, 95.9115) centre (-34.2688, 73.203) ccw
sketch "Sketch16" plane through (0, -27.5, 0) normal (0, -1, 0) x (1, 0, 0)
  line L0 (-20.7688, 96.5857) -> (-20.7688, 77.5857)
  arc A0 (-47.7688, 77.5857) -> (-20.7688, 77.5857) centre (-34.2688, 100.9684) ccw
  line L1 (-47.7688, 77.5857) -> (-47.7688, 96.5857)
  arc A1 (-20.7688, 96.5857) -> (-47.7688, 96.5857) centre (-34.2688, 73.203) ccw
  circle A2 centre (-190.7032, 183.5) radius 3
  circle A3 centre (-190.7032, 136.5) radius 3
  circle A4 centre (-150, 113) radius 3
  circle A5 centre (-109.2968, 136.5) radius 3
  circle A6 centre (-109.2968, 183.5) radius 3
  circle A7 centre (-150, 207) radius 3
  arc A8 (-133.1676, 207.0815) -> (-141.0365, 209.19) centre (-150, 160) ccw
  arc A9 (-133.1676, 207.0815) -> (-117.6424, 198.118) centre (-125, 203.3013) ccw
  arc A10 (-111.8819, 192.3576) -> (-117.6424, 198.1181) centre (-150, 160) ccw
  arc A11 (-111.8819, 192.3576) -> (-102.9185, 176.8324) centre (-106.6987, 185) ccw
  arc A12 (-100.81, 168.9635) -> (-102.9185, 176.8324) centre (-150, 160) ccw
  arc A13 (-100.81, 168.9635) -> (-100.81, 151.0365) centre (-100, 160) ccw
  arc A14 (-102.9185, 143.1676) -> (-100.81, 151.0365) centre (-150, 160) ccw
  arc A15 (-102.9185, 143.1676) -> (-111.882, 127.6424) centre (-106.6987, 135) ccw
  arc A16 (-117.6424, 121.8819) -> (-111.8819, 127.6424) centre (-150, 160) ccw
  arc A17 (-117.6424, 121.8819) -> (-133.1676, 112.9185) centre (-125, 116.6987) ccw
  arc A18 (-141.0365, 110.81) -> (-133.1676, 112.9185) centre (-150, 160) ccw
  arc A19 (-141.0365, 110.81) -> (-158.9635, 110.81) centre (-150, 110) ccw
  arc A20 (-166.8324, 112.9185) -> (-158.9635, 110.81) centre (-150, 160) ccw
  arc A21 (-166.8324, 112.9185) -> (-182.3576, 121.882) centre (-175, 116.6987) ccw
  arc A22 (-188.1181, 127.6424) -> (-182.3576, 121.8819) centre (-150, 160) ccw
  arc A23 (-188.1181, 127.6424) -> (-197.0815, 143.1676) centre (-193.3013, 135) ccw
  arc A24 (-199.19, 151.0365) -> (-197.0815, 143.1676) centre (-150, 160) ccw
  arc A25 (-199.19, 151.0365) -> (-199.19, 168.9635) centre (-200, 160) ccw
  arc A26 (-197.0815, 176.8324) -> (-199.19, 168.9635) centre (-150, 160) ccw
  arc A27 (-197.0815, 176.8324) -> (-188.118, 192.3576) centre (-193.3013, 185) ccw
  arc A28 (-182.3576, 198.1181) -> (-188.1181, 192.3576) centre (-150, 160) ccw
  arc A29 (-182.3576, 198.1181) -> (-166.8324, 207.0815) centre (-175, 203.3013) ccw
  arc A30 (-158.9635, 209.19) -> (-166.8324, 207.0815) centre (-150, 160) ccw
  arc A31 (-158.9635, 209.19) -> (-141.0365, 209.19) centre (-150, 210) ccw
  arc A32 (-103.8359, 194.7625) -> (-157.0151, 102.6385) centre (-150, 160) ccw
  arc A33 (-72.4228, 58.5017) -> (-157.0151, 102.6385) centre (-173.4894, -32.069) ccw
  arc A34 (-72.4228, 58.5017) -> (14.1053, 85.7195) centre (-68.6761, 197.7402) ccw
  arc A35 (-103.8359, 194.7625) -> (14.1053, 85.7195) centre (256.2101, 465.8849) ccw
  circle A36 centre (-126.5, 200.7032) radius 3
  circle A37 centre (-103, 160) radius 3
  circle A38 centre (-126.5, 119.2968) radius 3
  circle A39 centre (-173.5, 119.2968) radius 3
  circle A40 centre (-197, 160) radius 3
  circle A41 centre (-173.5, 200.7032) radius 3
  line L2 (-47.7688, 77.5857) -> (-20.7688, 96.5857)
  circle A42 centre (-34.2688, 87.0857) radius 17.857
  circle A43 centre (-34.2688, 87.0857) radius 19.1735
  circle A44 centre (-71.2492, 87.0857) radius 6.5
  circle A45 centre (-71.2492, 87.0857) radius 3.5
  dimension "d61" = 35.714
  dimension "d62" = 38.347
  dimension "d63" = 13
  dimension "d64" = 7
  constraint coincident L0.start A1.start
  constraint coincident A0.start L1.start
  constraint midpoint L2 A42.centre
  constraint concentric A42 A43
  constraint concentric A44 A45
  measures "d61" diameter of A42
  measures "d62" diameter of A43
  measures "d63" diameter of A44
  measures "d64" diameter of A45
extrude "Extrude15" cut sketch "Sketch16" against normal blind 0.9 contours A43 | A44 in component "Component"
sketch "Sketch17" plane through (0, 0, 0) normal (0, 0, 1) x (1, 0, 0)
  circle A0 centre (0, 0) radius 15
  dimension "d67" = 30
  constraint coincident A0.centre origin
  measures "d67" diameter of A0
extrude "Extrude16" cut sketch "Sketch17" along normal blind 20 in component "Component"
fillet "Fillet1" radius 4 10 edges at (77.5, 20, 62) (55, 20, 87) (-113.7109, 20, 77.7105) (-209.3252, 20, 194.2458) (-37.0038, 20, 137.8215) (77.5, 0, 87) (77.5, -20, 62) (55, -20, 87) (-77.5, -20, 42.5) (-77.5, 20, 42.5) in component "Component"
sketch "Sketch18" plane through (0, 20, 0) normal (0, 1, 0) x (-1, 0, 0)
  line L0 (-73.5, 83) -> (-73.5, 37)
  line L1 (-73.5, 37) -> (73.5, 37)
  line L2 (73.5, 37) -> (73.5, 49.4364)
  arc A0 (157.8298, 95.977) -> (73.5, 49.4364) centre (173.4894, -32.069) ccw
  arc A1 (157.8298, 95.977) -> (98.4748, 198.7996) centre (150, 160) ccw
  arc A2 (-31.4099, 83) -> (98.4748, 198.7996) centre (-256.2101, 465.8849) ccw
  line L3 (-31.4099, 83) -> (-73.5, 83)
  circle A3 centre (150, 160) radius 15
  dimension "d72" = 30
  constraint concentric A1 A3
  measures "d72" diameter of A3
extrude "Extrude17" cut sketch "Sketch18" against normal blind 20 contours A3 in component "Component"
component "Component" placed x (1, 0, 0) y (0, 1, 0) z (0, 0, 1) at (0, 0, 0)

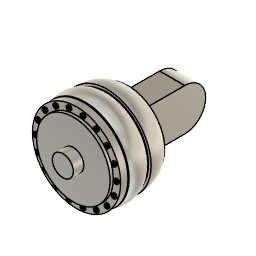
design "industrial bot"
part number: 2025-10-27-23-58-21-680
Autodesk Fusion 360 part; units mm, degrees
sketch "Sketch1" plane through (0, 0, 0) normal (0, 0, 1) x (1, 0, 0)
  line L0 (0, 0) -> (-35, 0)
  line L1 (0, 0) -> (0, -20)
  line L2 (0, -20) -> (-42, -20)
  arc A0 (-35, 0) -> (-42, -20) centre (-17.1273, -17.4804) ccw
  dimension "d1" = 35
  dimension "d2" = 20
  dimension "d3" = 42
  dimension "d4" = 25
  constraint coincident L0.start L1.start
  constraint horizontal L0
  constraint perpendicular L0 L1
  constraint perpendicular L1 L2
  measures "d1" distance of L0.start L0.end
  measures "d2" distance of L0.start L1.end
  measures "d3" distance of L1.end L2.end
  measures "d4" radius of A0
revolve "Revolve1" add sketch "Sketch1" angle 360 about axis through (0, 0, 0) along (0, -1, 0) makes body 1
sketch "Sketch2" plane through (0, -20, 0) normal (0, -1, 0) x (1, 0, 0)
  circle A0 centre (0, 0) radius 42
  circle A1 centre (0, 0) radius 39.5
  dimension "d6" = 79
  constraint coincident A0.centre A1.centre
  measures "d6" diameter of A1
extrude "Extrude1" add sketch "Sketch2" along normal blind 1 contours A1 bodies 1
sketch "Sketch3" plane through (0, 0, 0) normal (0, 0, 1) x (1, 0, 0)
  line L0 (0, -21) -> (0, -41)
  line L1 (0, -41) -> (-42, -41)
  line L2 (0, -21) -> (-40, -21)
  arc A0 (-40, -21) -> (-42, -41) centre (-23.7942, -32.7206) ccw
  dimension "d9" = 20
  dimension "d10" = 42
  dimension "d11" = 40
  dimension "d12" = 20
  constraint vertical L0
  constraint perpendicular L0 L1
  constraint perpendicular L0 L2
  measures "d9" distance of L0.start L0.end
  measures "d10" distance of L0.end L1.end
  measures "d11" distance of L0.start L2.end
  measures "d12" radius of A0
revolve "Revolve2" add sketch "Sketch3" angle 360 about axis through (0, -21, 0) along (0, -1, 0) bodies 1
sketch "Sketch4" plane through (0, -41, 0) normal (0, -1, 0) x (1, 0, 0)
  circle A0 centre (0, 0) radius 42
  circle A1 centre (0, 0) radius 41.25
  dimension "d14" = 82.5
  constraint coincident A0.centre A1.centre
  measures "d14" diameter of A1
extrude "Extrude2" add sketch "Sketch4" along normal blind 1 contours A1 bodies 1
sketch "Sketch5" plane through (0, -42, 0) normal (0, -1, 0) x (1, 0, 0)
  circle A0 centre (0, 0) radius 41.25
  circle A1 centre (0, 0) radius 42
  dimension "d17" = 84
  constraint coincident A0.centre A1.centre
  measures "d17" diameter of A1
extrude "Extrude3" add sketch "Sketch5" along normal blind 7 contours A0 | A1 bodies 1
sketch "Sketch6" plane through (0, -49, 0) normal (0, -1, 0) x (1, 0, 0)
  circle A0 centre (0, 0) radius 42
  circle A1 centre (0, 0) radius 35
  dimension "d20" = 70
  constraint coincident A0.centre A1.centre
  measures "d20" diameter of A1
extrude "Extrude4" add sketch "Sketch6" along normal blind 3 contours A1 bodies 1
sketch "Sketch7" plane through (0, -52, 0) normal (0, -1, 0) x (1, 0, 0)
  circle A0 centre (0, 0) radius 35
  line L0 (0, 0) -> (35, 0)
  line L1 (35, 0) -> (42, 0)
  circle A1 centre (38.5, 0) radius 2.25
  circle A2 centre (38.5, 0) radius 1.5
  dimension "d23" = 4.5
  dimension "d24" = 3
  constraint coincident A0.centre L0.start
  constraint coincident A0 L0.end
  constraint horizontal L0
  constraint parallel L0 L1
  constraint midpoint L1 A1.centre
  constraint concentric A1 A2
  measures "d23" diameter of A1
  measures "d24" diameter of A2
extrude "Extrude5" add sketch "Sketch7" along normal blind 1 separate body contours L1 A1 A2 | L1 A1 A2 makes body 2
pattern_circular "C-Pattern1" count 18 over 360 about axis through (0, -49, 0) along (0, 1, 0) of "Extrude5" makes body 3 at (34.3756, -52, -12.3134) makes body 4 at (28.0389, -52, -23.3815) makes body 5 at (18.4183, -52, -31.5289) makes body 6 at (6.5241, -52, -35.9269) makes body 7 at (-6.1571, -52, -35.9916) makes body 8 at (-18.0956, -52, -31.7152) makes body 9 at (-27.8952, -52, -23.5528) makes body 10 at (-34.2482, -52, -12.6636) makes body 11 at (-36.514, -52, -0.1863) makes body 12 at (-34.3756, -52, 12.3134) makes body 13 at (-28.0389, -52, 23.3815) makes body 14 at (-18.4183, -52, 31.5289) makes body 15 at (-6.5241, -52, 35.9269) makes body 16 at (6.1571, -52, 35.9916) makes body 17 at (18.0956, -52, 31.7152) makes body 18 at (27.8952, -52, 23.5528) makes body 19 at (34.2482, -52, 12.6636)
sketch "Sketch8" plane through (0, 0, 0) normal (0, 1, 0) x (-1, 0, 0)
  circle A0 centre (0, 0) radius 35
  line L0 (12, 20) -> (-12, 20)
  line L1 (-12, 20) -> (-12, -20)
  line L2 (-12, -20) -> (12, -20)
  line L3 (12, -20) -> (12, 20)
  line L4 (12, 20) -> (-12, -20) construction
  line L5 (-12, 20) -> (12, -20) construction
  dimension "d29" = 24
  dimension "d30" = 40
  constraint horizontal L0
  constraint perpendicular L0 L1
  constraint parallel L0 L2
  constraint parallel L1 L3
  constraint coincident L4 A0.centre
  constraint coincident L5 A0.centre
  constraint coincident A0.centre origin
  measures "d29" distance of L0.start L0.end
  measures "d30" distance of L0.start L2.end
extrude "Extrude6" add sketch "Sketch8" along normal blind 42 contours L0 L1 L2 L3 bodies 1
sketch "Sketch9" plane through (-12, 0, 0) normal (-1, 0, 0) x (0, -1, 0)
  line L0 (0, -20) -> (0, 20)
  line L1 (0, 20) -> (-42, 20)
  line L2 (-42, 20) -> (-42, -20)
  line L3 (-42, -20) -> (0, -20)
  circle A0 centre (-42, 0) radius 20
  constraint midpoint L2 A0.centre
  constraint coincident L1.end A0
extrude "Extrude7" add sketch "Sketch9" against normal blind 24 contours L2 A0 picked at (-48.2058, 2.4356) bodies 1
sketch "Sketch10" plane through (-12, 0, 0) normal (-1, 0, 0) x (0, -1, 0)
  line L0 (0, -20) -> (0, 20)
  line L1 (0, 20) -> (-42, 20)
  arc A0 (-42, 20) -> (-42, -20) centre (-42, 0) ccw
  line L2 (-42, -20) -> (0, -20)
  circle A1 centre (-42, 0) radius 10
  dimension "d35" = 20
  constraint concentric A0 A1
  measures "d35" diameter of A1
extrude "Extrude8" add sketch "Sketch10" along normal blind 10 contours A1 bodies 1
sketch "Sketch11" plane through (0, -52, 0) normal (0, -1, 0) x (1, 0, 0)
  circle A0 centre (0, 0) radius 35
  circle A1 centre (0, 0) radius 10
  dimension "d38" = 20
  constraint coincident A0.centre A1.centre
  measures "d38" diameter of A1
extrude "Extrude9" add sketch "Sketch11" along normal blind 10 contours A1 bodies 1
move_body "Move1" bodies 2 3 4 5 6 7 8 9 10 11 12 13 14 15 16 17 18 19 to x (1, 0, 0) y (0, 1, 0) z (0, 0, 1) at (0, 0.1365, 0.0409)
move_body "Move2" bodies 2 3 4 5 6 7 8 9 10 11 12 13 14 15 16 17 18 19 to x (1, 0, 0) y (0, 1, 0) z (0, 0, 1) at (0, 3, 0)
move_body "Move3" bodies 2 3 4 5 6 7 8 9 10 11 12 13 14 15 16 17 18 19 to x (1, 0, 0) y (0, 1, 0) z (0, 0, 1) at (0, -0.1, 0)
